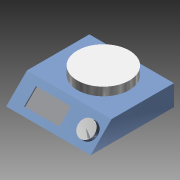
# Autodesk Inventor part: hotplate
Saved by Autodesk Inventor 2014 (Build 180170000, 170)
## iProperties
Created: 2014-07-14
Part Number: hotplate
Material: Generic
Document SubType Name: Modeling
Designer: Nabeel
Density: 1 g/cm^3
Appearance: Default
Author: Nabeel
Autodesk Inventor part; units mm, degrees
ref_plane "YZ Plane" through (0, 0, 0) normal (1, 0, 0) x (0, 1, 0)
ref_plane "XZ Plane" through (0, 0, 0) normal (0, 1, 0) x (-1, 0, 0)
ref_plane "XY Plane" through (0, 0, 0) normal (0, 0, 1) x (1, 0, 0)
sketch "Sketch1" plane through (0, 0, 0) normal (0, 0, 1) x (1, 0, 0)
  line L0 (-40.6, 0) -> (243.6, 0) projected
  line L1 (0, -40) -> (0, 240) projected
  line L2 (0, 0) -> (203, 0)
  line L3 (203, 0) -> (203, 200)
  line L4 (203, 200) -> (0, 200)
  line L5 (0, 200) -> (0, 0)
  dimension "d0" = 203
  dimension "d1" = 200
  constraints: 8 end point, 2 parallel, 1 horizontal, 1 perpendicular
  measures "d0" distance between parallel lines of L3 L5
  measures "d1" distance between parallel lines of L4 L2
extrude "Extrusion1" add sketch "Sketch1" along normal blind 50
sketch "Sketch2" plane through (0, 0, 50) normal (0, 0, 1) x (1, 0, 0)
  circle A0 centre (101.5, 132.0548) radius 62.5
  dimension "d4" = 125
  constraints: 1 centre point
  measures "d4" diameter of A0
extrude "Extrusion2" add sketch "Sketch2" along normal blind 20
chamfer "Chamfer1" distance 50 angle 45 1 edges at (101.5, 0, 50)
sketch "Sketch3" plane through (0, 50, 50) normal (0, -0.7071068, 0.7071068) x (1, 0, 0)
  circle A0 centre (175.1245, -35.3553) radius 20
  dimension "d10" = 40
  constraints: 1 centre point
  measures "d10" diameter of A0
extrude "Extrusion3" add sketch "Sketch3" along normal blind 10
sketch "Sketch4" plane through (0, 50, 50) normal (0, -0.7071068, 0.7071068) x (1, 0, 0)
  line L0 (32.6771, -55.3553) -> (116.9718, -55.3553)
  line L1 (116.9718, -55.3553) -> (116.9718, -15.3553)
  line L2 (116.9718, -15.3553) -> (32.6771, -15.3553)
  line L3 (32.6771, -15.3553) -> (32.6771, -55.3553)
  constraints: 8 end point, 2 parallel, 1 horizontal, 1 perpendicular
extrude "Extrusion4" cut sketch "Sketch4" against normal blind 3
sketch "Sketch6" plane through (175.1245, 17.9289, 32.0711) normal (0, -0.7071068, 0.7071068) x (1, 0, 0)
  circle A0 centre (0, 0) radius 20 projected
  line L0 (0, 0) -> (14.6725, -8.8501)
  line L1 (0, 0) -> (12.4199, -12.5846)
  arc A1 (12.4199, -12.5846) -> (14.6725, -8.8501) centre (12.5538, -10.1188) ccw
  point P0 (-175.1245, -35.3553)
  constraints: 4 end point, 2 point on circle, 1 centre point
extrude "Extrusion5" add sketch "Sketch6" along normal blind 1.5 contours L0 A1 L1
thread "Thread1" size "M42x1.5" standard "Din Taper" length 10
body "Solid1"
